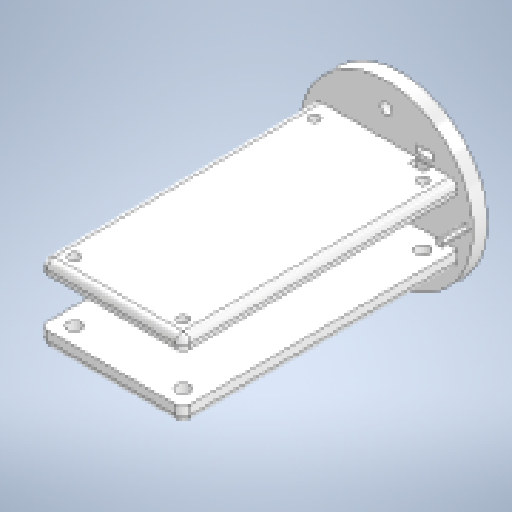
# Autodesk Inventor part: Supportv2_3dprinted
Saved by Autodesk Inventor 2023 (Build 270158000, 158)
## iProperties
Created: 2022-10-05
Part Number: Supportv2_3dprinted
Material: ABS Plastic
Document SubType Name: Modeling
Designer: jeanp
Density: 1.06 g/cm^3
Appearance: Smooth - White
Author: jeanp
Autodesk Inventor part; units mm, degrees
ref_plane "YZ Plane" through (0, 0, 0) normal (1, 0, 0) x (0, 1, 0)
ref_plane "XZ Plane" through (0, 0, 0) normal (0, 1, 0) x (-1, 0, 0)
ref_plane "XY Plane" through (0, 0, 0) normal (0, 0, 1) x (1, 0, 0)
sketch "Sketch1" plane through (0, 0, 0) normal (0, 0, 1) x (1, 0, 0)
  circle A0 centre (0, 0) radius 37.7825
  dimension "d0" = 75.565
  constraints: 1 centre point, 1 coincident
  measures "d0" diameter of A0
extrude "Extrusion1" add sketch "Sketch1" against normal blind 6.35
sketch "Sketch2" plane through (0, 0, 0) normal (0, 0, 1) x (1, 0, 0)
  line L0 (-31.115, -10.4775) -> (31.115, -10.4775)
  line L1 (31.115, -10.4775) -> (31.115, -17.6657)
  line L2 (31.115, -17.6657) -> (-31.115, -17.6657)
  line L3 (-31.115, -17.6657) -> (-31.115, -10.4775)
  line L4 (-31.115, 15.5575) -> (31.115, 15.5575)
  line L5 (31.115, 15.5575) -> (31.115, 10.4775)
  line L6 (31.115, 10.4775) -> (-31.115, 10.4775)
  line L7 (-31.115, 10.4775) -> (-31.115, 15.5575)
  point P0 (0, 0)
  point P1 (31.115, -14.0716)
  point P2 (31.115, 13.0175)
  dimension "d3" = 7.1882
  dimension "d4" = 62.23
  dimension "d5" = 31.115
  dimension "d6" = 10.4775
  dimension "d10" = 62.23
  dimension "d11" = 31.115
  dimension "d12" = 10.4775
  dimension "d13" = 5.08
  constraints: 16 end point, 4 parallel, 2 horizontal, 2 midpoint, 2 perpendicular
  measures "d3" distance of L2.end L0.start
  measures "d4" distance of L0.start L0.end
  measures "d5" horizontal distance of point (0, 0) point (31.115, -14.072)
  measures "d6" distance from line of L0 point (0, 0)
  measures "d10" distance of L4.start L4.end
  measures "d11" horizontal distance of point (0, 0) point (31.115, 13.018)
  measures "d12" distance from line of L6 point (0, 0)
  measures "d13" distance between parallel lines of L4 L6
extrude "Extrusion2" add sketch "Sketch2" along normal blind 119.38
fillet "Fillet1" radius 3.175 5 edges at (-31.115, -14.0716, 119.38) (31.115, -14.0716, 119.38) (31.115, -17.6657, 59.69) (-31.115, -17.6657, 59.69) (0, -17.6657, 119.38)
fillet "Fillet2" radius 3.175 5 edges at (-31.115, 13.0175, 119.38) (31.115, 13.0175, 119.38) (-31.115, 15.5575, 59.69) (0, 15.5575, 119.38) (31.115, 15.5575, 59.69)
sketch "Sketch3" plane through (-31.115, -10.4775, 0) normal (0, 1, 0) x (1, 0, 0)
  line L0 (0, -116.205) -> (0, 0) projected
  line L1 (59.055, -119.38) -> (3.175, -119.38) projected
  line L2 (62.23, 0) -> (62.23, -116.205) projected
  line L3 (59.055, 0) -> (3.175, 0) projected
  point P0 (31.115, 0)
  point P1 (7.5438, -111.8362)
  point P2 (7.5438, -7.5438)
  point P3 (54.6862, -7.5438)
  point P4 (54.6862, -111.8362)
  dimension "d15" = 7.5438
  dimension "d16" = 7.5438
  dimension "d17" = 7.5438
  dimension "d18" = 7.5438
  dimension "d19" = 7.5438
  dimension "d20" = 7.5438
  dimension "d21" = 7.5438
  dimension "d22" = 7.5438
  measures "d15" distance from line of L0 point (7.544, -111.836)
  measures "d16" distance from line of point (7.544, -111.836) L1
  measures "d17" distance from line of point (54.686, -111.836) L2
  measures "d18" distance from line of L1 point (54.686, -111.836)
  measures "d19" distance from line of point (54.686, -7.544) L2
  measures "d20" distance from line of point (54.686, -7.544) L3
  measures "d21" distance from line of L0 point (7.544, -7.544)
  measures "d22" distance from line of point (7.544, -7.544) L3
hole "Hole1" at (-23.5712, -10.4775, 111.8362) at (-23.5712, -10.4775, 7.5438) at (23.5712, -10.4775, 7.5438) at (23.5712, -10.4775, 111.8362) direction (0, -1, 0) diameter 5.842 end through all
sketch "Sketch4" plane through (-31.115, 10.4775, 0) normal (0, -1, 0) x (1, 0, 0)
  circle A0 centre (54.6862, 111.8362) radius 2.1717 projected
  circle A1 centre (54.6862, 7.5362) radius 2.1717 projected
  circle A2 centre (7.5362, 7.5362) radius 2.1717 projected
  circle A3 centre (7.5362, 111.8362) radius 2.1717 projected
  point P0 (31.115, 0)
hole "Hole2" at (23.5712, 10.4775, 111.8362) at (-23.5788, 10.4775, 111.8362) at (-23.5788, 10.4775, 7.5362) at (23.5712, 10.4775, 7.5362) direction (0, 1, 0) diameter 4.4958 end through all clearance for "Flat Head Machine Screw (82)" size "#8" standard "Ansi Unified Screw Threads"
sketch "Sketch5" plane through (0, 0, -6.35) normal (0, 0, -1) x (-1, 0, 0)
  circle A0 centre (0, 27.305) radius 2.921 projected
  arc A1 (-0.6096, -25.2301) -> (-0.6096, -29.3799) centre (0, -27.305) ccw projected
  point P0 (0, 0)
hole "Hole3" at (0, 27.305, -6.35) at (0, -27.305, -6.35) direction (0, 0, 1) diameter 4.4958 end through all clearance for "Flat Head Machine Screw (82)" size "#8" standard "Ansi Unified Screw Threads"
sketch "Sketch7" plane through (0, 0, -6.35) normal (0, 0, -1) x (-1, 0, 0)
  line L0 (21.939, 20) -> (25.939, 20)
  line L1 (25.939, 20) -> (25.939, -20)
  line L2 (25.939, -20) -> (21.939, -20)
  line L3 (21.939, -20) -> (21.939, 20)
  line L4 (22.439, -16.8541) -> (22.439, 16.8541) projected
  line L5 (25.439, 16.8541) -> (25.439, -16.8541) projected
  point P0 (0, 0)
  point P1 (23.939, -20)
  point P2 (23.939, 20)
  dimension "d51" = 4
  dimension "d53" = 0.5
  dimension "d54" = 40
  dimension "d55" = 20
  constraints: 8 end point, 2 midpoint, 2 parallel, 1 horizontal, 1 perpendicular
  measures "d51" distance between parallel lines of L1 L3
  measures "d53" distance between parallel lines of L3 L4
  measures "d54" distance of point (23.939, -20) point (23.939, 20)
  measures "d55" vertical distance of point (23.939, 20) point (0, 0)
extrude "Extrusion4" cut sketch "Sketch7" against normal blind 3
sketch "Sketch8" plane through (0, 0, -6.35) normal (0, 0, -1) x (-1, 0, 0)
  line L0 (27.94, 15.5575) -> (-27.94, 15.5575) projected
  line L1 (-20.1422, 20.5105) -> (-13.7922, 20.5105)
  line L2 (-13.7922, 20.5105) -> (-13.7922, 17.3355)
  line L3 (-13.7922, 17.3355) -> (-20.1422, 17.3355)
  line L4 (-20.1422, 17.3355) -> (-20.1422, 20.5105)
  line L5 (-20.1422, 20.3225) -> (-20.1422, 16.7818)
  point P0 (0, 0)
  dimension "d58" = 6.35
  dimension "d59" = 3.175
  dimension "d60" = 0
  dimension "d61" = 1.778
  constraints: 10 end point, 2 parallel, 1 horizontal, 1 perpendicular, 1 vertical, 2 other
  measures "d58" distance of L1.start L1.end
  measures "d59" distance of L1.end L2.end
  measures "d60" distance between parallel lines of L5 L4
  measures "d61" distance between parallel lines of L0 L3
extrude "Extrusion5" cut sketch "Sketch8" against normal through all
sketch "Sketch9" plane through (-27.94, 15.5575, 0) normal (0, 1, 0) x (1, 0, 0)
  line L0 (41.7322, -0.635) -> (48.0822, -0.635)
  line L1 (48.0822, -0.635) -> (48.0822, -3.81)
  line L2 (48.0822, -3.81) -> (41.7322, -3.81)
  line L3 (41.7322, -3.81) -> (41.7322, -0.635)
  line L4 (-9.8425, 0) -> (65.7225, 0) projected
  point P0 (27.94, 0)
  point P1 (41.7322, 0)
  point P2 (48.0822, 0)
  point P3 (48.0822, -2.2225)
  dimension "d64" = 0
  dimension "d66" = 0
  dimension "d67" = 0.635
  dimension "d68" = 3.175
  constraints: 8 end point, 2 parallel, 1 horizontal, 1 midpoint, 1 perpendicular
  measures "d64" distance from line of point (41.732, 0) L3
  measures "d66" distance from line of point (48.082, 0) L1
  measures "d67" distance between parallel lines of L4 L0
  measures "d68" distance between parallel lines of L0 L2
extrude "Extrusion6" cut sketch "Sketch9" against normal up to next
sketch "Sketch10" plane through (0, 0, 0) normal (0, 0, 1) x (1, 0, 0)
  line L0 (33.2105, 1.5875) -> (36.3855, 1.5875)
  line L1 (36.3855, 1.5875) -> (36.3855, -1.5875)
  line L2 (36.3855, -1.5875) -> (33.2105, -1.5875)
  line L3 (33.2105, -1.5875) -> (33.2105, 1.5875)
  circle A0 centre (0, 0) radius 37.7825 projected
  line L4 (36.2585, 1.4605) -> (33.3375, 1.4605)
  line L5 (33.3375, 1.4605) -> (33.3375, -1.4605)
  line L6 (33.3375, -1.4605) -> (36.2585, -1.4605)
  line L7 (36.2585, -1.4605) -> (36.2585, 1.4605)
  dimension "d71" = 3.175
  dimension "d72" = 3.175
  dimension "d73" = 36.3855
  dimension "d74" = 37.7825
  dimension "d75" = 0.127
  dimension "d79" = 1.5875
  constraints: 16 end point, 4 parallel, 2 perpendicular, 1 horizontal, 3 other
  measures "d71" distance of L0.start L0.end
  measures "d72" distance of L0.end L1.end
  measures "d73" distance from line of L1 A0.centre
  measures "d74" radius of A0
  measures "d75" distance between parallel lines of L0 L4
  measures "d79" distance from line of point (0, 0) L2
extrude "Extrusion7" add sketch "Sketch10" along normal blind 6.35 contours L7 L6 L5 L4
fillet "Fillet4" radius 1 4 edges at (33.3375, 1.4605, 3.175) (36.2585, 1.4605, 3.175) (36.2585, -1.4605, 3.175) (33.3375, -1.4605, 3.175)
equation "\"d5\" = 0.5 * d4"
equation "\"d10\" = d4"
equation "\"d11\" = 0.5 * d10"
equation "\"d12\" = d6"
equation "\"d16\" = d15"
equation "\"d17\" = d16"
equation "\"d18\" = d16"
equation "\"d19\" = d17"
equation "\"d20\" = d19"
equation "\"d21\" = d15"
equation "\"d22\" = d21"
body "Solid1"
